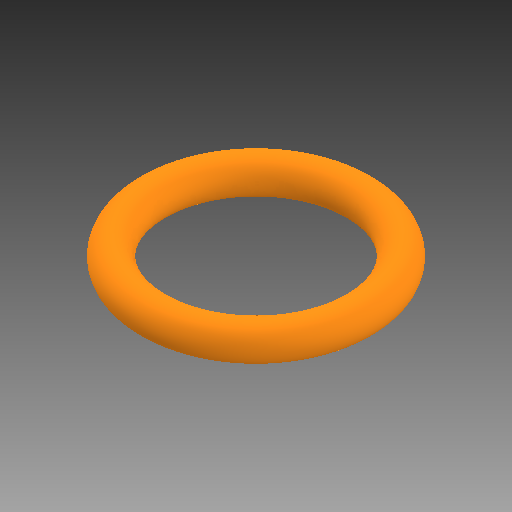
# Autodesk Inventor part: 2024 Note
Saved by Autodesk Inventor 2025 (Build 290162000, 162)
## iProperties
Created: 2024-07-19
Part Number: 2024 Note
Material: Generic
Document SubType Name: Modeling
Designer: Minotaur
Density: 1 g/cm^3
Appearance: Orange
Author: Minotaur
Autodesk Inventor part; units mm, degrees
ref_plane "YZ Plane" through (0, 0, 0) normal (1, 0, 0) x (0, 1, 0)
ref_plane "XZ Plane" through (0, 0, 0) normal (0, 1, 0) x (-1, 0, 0)
ref_plane "XY Plane" through (0, 0, 0) normal (0, 0, 1) x (1, 0, 0)
sketch "Sketch1" plane through (0, 0, 0) normal (0, 0, 1) x (1, 0, 0)
  circle A0 centre (-152.4, 0) radius 25.4
  line L0 (0, 0) -> (0, 33.1048) construction
  point P0 (-177.8, 0)
  dimension "d0" = 254
  dimension "d1" = 355.6
  constraints: 3 horizontal alignment, 2 end point, 1 vertical, 2 other
  measures "d1" diameter of point (-177.8, 0) L0
revolve "Revolution1" add sketch "Sketch1" angle 360 about axis through (0, 0, 0) along (0, 1, 0)
body "Solid1"
